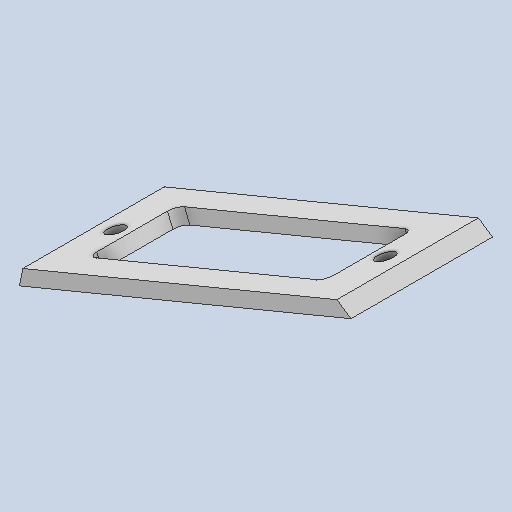
# Autodesk Inventor part: ДМФ 0124 Нижний лист
Saved by Autodesk Inventor 2024.2 (Build 282272000, 272)
## iProperties
Created: 2024-05-05
Part Number: ДМФ 0124 Нижний лист
Material: Generic
Document SubType Name: Modeling
Designer: pokla
Density: 1 g/cm^3
Appearance: Default
Author: pokla
Autodesk Inventor part; units mm, degrees
ref_plane "YZ Plane" through (0, 0, 0) normal (1, 0, 0) x (0, 1, 0)
ref_plane "XZ Plane" through (0, 0, 0) normal (0, 1, 0) x (-1, 0, 0)
ref_plane "XY Plane" through (0, 0, 0) normal (0, 0, 1) x (1, 0, 0)
sketch "Sketch2" plane through (0, 0, 0) normal (0, 0, 1) x (1, 0, 0)
  line L0 (0, 273.8452) -> (193.6378, 193.6378) construction
  line L1 (193.6378, 193.6378) -> (273.8452, 0) construction
  line L2 (273.8452, 0) -> (193.6378, -193.6378) construction
  line L3 (193.6378, -193.6378) -> (0, -273.8452) construction
  line L4 (0, -273.8452) -> (-193.6378, -193.6378) construction
  line L5 (-193.6378, -193.6378) -> (-273.8452, 0) construction
  line L6 (-273.8452, 0) -> (-193.6378, 193.6378) construction
  line L7 (-193.6378, 193.6378) -> (0, 273.8452) construction
  line L8 (-193.6378, 193.6378) -> (0, 273.8452) construction
  line L9 (-459.9272, 770.6562) -> (-219.7185, 870.1539) construction
  line L10 (-96.8189, 233.7415) -> (-339.8229, 820.405) construction
  line L11 (-219.7185, 870.1539) -> (0, 870.1539) construction
  line L12 (0, 870.1539) -> (0, 273.8452) construction
  line L13 (-459.9272, 770.6562) -> (-615.2917, 615.2917) construction
  line L14 (-615.2917, 615.2917) -> (-193.6378, 193.6378) construction
  line L15 (-5, 277.1861) -> (-192.4647, 199.5357) construction
  line L16 (-192.4647, 199.5357) -> (-608.2206, 615.2917) construction
  line L17 (-608.2206, 615.2917) -> (-457.095, 766.4174) construction
  line L18 (-457.095, 766.4174) -> (-218.724, 865.1539) construction
  line L19 (-218.724, 865.1539) -> (-5, 865.1539) construction
  line L20 (-5, 865.1539) -> (-5, 277.1861) construction
  line L21 (-13, 282.5315) -> (-190.5876, 208.9724) construction
  line L22 (-190.5876, 208.9724) -> (-596.9069, 615.2917) construction
  line L23 (-596.9069, 615.2917) -> (-452.5633, 759.6353) construction
  line L24 (-452.5633, 759.6353) -> (-217.1327, 857.1539) construction
  line L25 (-217.1327, 857.1539) -> (-13, 857.1539) construction
  line L26 (-13, 857.1539) -> (-13, 282.5315) construction
  line L27 (-5, 277.1861) -> (-192.4647, 199.5357)
  line L28 (-192.4647, 199.5357) -> (-190.5876, 208.9724)
  line L29 (-190.5876, 208.9724) -> (-13, 282.5315)
  line L30 (-13, 282.5315) -> (-5, 277.1861)
  point P0 (0, 0)
  point P1 (0, 0)
  point P2 (0, 0)
  dimension "d0" = 506
  dimension "d1" = 260
  dimension "d2" = 635
  dimension "d6" = 5
  dimension "d7" = 8
  constraints: 62 end point, 2 coincident, 2 midpoint, 2 parallel, 1 horizontal, 1 perpendicular, 1 symmetric about line, 1 vertical, 1 vertical alignment, 27 other
  measures "d0" distance between parallel lines of L5 L1
  measures "d1" distance of L9.start L11.start
  measures "d2" distance of L10.end L10.start
  measures "d6" distance between parallel lines of L12 L20
  measures "d7" distance between parallel lines of L20 L26
extrude "Extrusion1" add sketch "Sketch2" along normal mid plane 80
sketch "Sketch3" plane through (-13, 282.5315, -40) normal (-0.3827, 0.9239, 0) x (0.9239, 0.3827, 0)
  line L0 (-168.6097, -15) -> (-23.6097, -15)
  line L1 (-23.6097, -15) -> (-23.6097, -65)
  line L2 (-23.6097, -65) -> (-168.6097, -65)
  line L3 (-168.6097, -65) -> (-168.6097, -15)
  circle A0 centre (-13.6097, -40) radius 5
  circle A1 centre (-178.6097, -40) radius 5
  line L4 (0, -80) -> (-192.2194, -80) projected
  line L5 (-96.1097, -40) -> (-96.1097, -80) construction
  line L6 (5.3454, 0) -> (5.3454, -80) construction
  point P0 (-96.1097, -15)
  point P1 (-168.6097, -40)
  point P2 (-23.6097, -40)
  point P3 (5.3454, -40)
  dimension "d10" = 145
  dimension "d11" = 10
  dimension "d12" = 10
  dimension "d13" = 50
  constraints: 10 end point, 5 midpoint, 3 horizontal alignment, 2 centre point, 2 parallel, 2 perpendicular, 1 equal radius, 1 horizontal, 1 vertical alignment, 1 other
  measures "d10" distance of L0.start L0.end
  measures "d11" diameter of A1
  measures "d12" distance of point (-168.61, -40) A1.centre
  measures "d13" distance of L0.end L1.end
extrude "Extrusion2" cut sketch "Sketch3" against normal up to surface (8 mm away)
fillet "Fillet1" radius 5 4 edges at (-167.2443, 214.3119, -25) (-33.2818, 269.801, -25) (-33.2818, 269.801, 25) (-167.2443, 214.3119, 25)
equation "\"d0\" = Барабан_габарит_по_кассетам"
equation "\"d1\" = Кассета_длина_грани"
equation "\"d2\" = Кассета_высота"
equation "\"d10\" = Длина_окна_барабан"
equation "\"d11\" = Диам_шпильки_под_кассету"
equation "\"d13\" = Ширина_окна_барабан"
equation "\"Барабан_габарит_по_кассетам\" = 506"
equation "\"Кассета_длина_грани\" = 260"
equation "\"Кассета_высота\" = 635"
equation "\"Длина_окна_барабан\" = 145"
equation "\"Диам_шпильки_под_кассету\" = 10"
equation "\"Ширина_окна_барабан\" = 50"
body "Solid1"
